screen holder_v3 (Autodesk Fusion 360 design; units mm, degrees)
Autodesk Fusion 360 part; units mm, degrees
sketch "Esquisse1" plane through (0, 0, 0) normal (0, 0, 1) x (1, 0, 0)
  line L0 (18, 11) -> (-18, 11)
  line L1 (-18, 11) -> (-18, -11)
  line L2 (-18, -11) -> (18, -11) construction
  line L3 (18, -11) -> (18, 11)
  line L4 (18, 11) -> (-18, -11) construction
  line L5 (-18, 11) -> (18, -11) construction
  line L6 (18, 17) -> (-18, 17)
  line L7 (-18, 17) -> (-18, -17)
  line L8 (-18, -17) -> (18, -17)
  line L9 (18, -17) -> (18, 17)
  line L10 (18, 17) -> (-18, -17) construction
  line L11 (-18, 17) -> (18, -17) construction
  line L12 (-20, -19) -> (20, -19)
  line L13 (20, -19) -> (20, 19)
  line L14 (20, 19) -> (-20, 19)
  line L15 (-20, 19) -> (-20, -19)
  line L16 (-18, -7) -> (18, -7)
  line L17 (-18, -17) -> (-20, -17)
  line L18 (18, -17) -> (20, -17)
  dimension "d1" = 36
  dimension "d2" = 22
  dimension "d3" = 36
  dimension "d4" = 34
  dimension "d5" = 2
  dimension "d6" = -4
  constraint horizontal L0
  constraint perpendicular L0 L1
  constraint parallel L0 L2
  constraint parallel L1 L3
  constraint coincident L4 origin
  constraint coincident L5 origin
  constraint horizontal L6
  constraint perpendicular L6 L7
  constraint parallel L6 L8
  constraint parallel L7 L9
  constraint coincident L10 origin
  constraint coincident L11 origin
  constraint coincident L15 L17.end
  constraint perpendicular L15 L17
  constraint coincident L13 L18.end
  constraint perpendicular L13 L18
  measures "d1" distance of L1.end L2.end
  measures "d2" distance of L0.end L1.end
  measures "d3" distance of L7.end L8.end
  measures "d4" distance of L6.start L8.end
extrude "Extrusion1" add sketch "Esquisse1" along normal blind 2 contours L1 L3 L6 L7 L9 L13 L14 L15 L17 L18 | L0 L6 L7 L9 | L1 L3 L7 L8 L9 L16 | L8 L12 L13 L15 L17 L18
extrude "Extrusion2" add sketch "Esquisse1" along normal blind 8 contours L1 L3 L6 L7 L9 L13 L14 L15 L17 L18 | L8 L12 L13 L15 L17 L18
extrude "Extrusion3" add sketch "Esquisse1" along normal blind 15 contours L8 L12 L13 L15 L17 L18
sketch "Esquisse2" plane through (0, -19, 0) normal (0, -1, 0) x (1, 0, 0)
  line L0 (-20, 0) -> (20, 0)
  line L1 (20, 0) -> (20, 15)
  line L2 (20, 15) -> (-20, 15)
  line L3 (-20, 15) -> (-20, 0)
  circle A0 centre (-15, 10) radius 1.7
  line L4 (0, 0) -> (0, 15) construction
  circle A1 centre (15, 10) radius 1.7
  dimension "d13" = 3.4
  dimension "d14" = 5
  dimension "d15" = 5
  constraint coincident L4.start origin
  constraint midpoint L2 L4.end
  constraint symmetric A0 L4 A1
  measures "d13" diameter of A0
  measures "d14" distance of L2 A0.centre
  measures "d15" distance of L3 A0.centre
fillet "Congé1" radius 10 2 edges at (-19, -17, 8) (19, -17, 8)
extrude "Extrusion4" cut sketch "Esquisse2" against normal through all contours A0 | A1
equation "d3 = d1"
equation "d11 = 5 mm + 10 mm"
